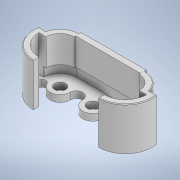
# Autodesk Inventor part: Real bottom
Saved by Autodesk Inventor 2020 (Build 240168000, 168)
## iProperties
Created: 2020-02-07
Part Number: Real bottom
Material: Generic
Document SubType Name: Modeling
Designer: Ball
Density: 1 g/cm^3
Appearance: Default
Author: Ball
Autodesk Inventor part; units mm, degrees
ref_plane "YZ Plane" through (0, 0, 0) normal (1, 0, 0) x (0, 1, 0)
ref_plane "XZ Plane" through (0, 0, 0) normal (0, 1, 0) x (-1, 0, 0)
ref_plane "XY Plane" through (0, 0, 0) normal (0, 0, 1) x (1, 0, 0)
sketch "Sketch1" plane through (0, 0, 0) normal (0, 1, 0) x (-1, 0, 0)
  line L0 (-25.6286, 14.9729) -> (-25.6286, 19.0115)
  line L1 (22.987, 19.0115) -> (22.987, 14.9729)
  arc A0 (-36.0426, -0.7751) -> (-25.6286, -11.1891) centre (-25.6286, -0.7751) ccw
  arc A1 (-39.8599, -4.3819) -> (-25.6286, -15.4563) centre (-25.6286, -0.7751) ccw
  line L2 (-25.6286, 14.9729) -> (-25.6286, 16.7446)
  arc A2 (22.987, -11.1891) -> (33.401, -0.7751) centre (22.987, -0.7751) ccw
  arc A3 (22.987, -15.4563) -> (37.2183, -4.3819) centre (22.987, -0.7751) ccw
  line L3 (22.987, 14.9729) -> (22.987, 16.7446)
  line L4 (-36.0426, -0.7751) -> (-41.3766, -0.7751)
  line L5 (-45.1939, -4.3446) -> (-45.1939, -4.3819)
  line L6 (-45.1939, -4.3819) -> (-39.8599, -4.3819)
  line L7 (33.401, -0.7751) -> (38.735, -0.7751)
  line L8 (42.5523, -4.3819) -> (37.2183, -4.3819)
  arc A4 (-25.6286, 14.9729) -> (-41.3766, -0.7751) centre (-25.6286, -0.7751) ccw
  line L9 (37.2183, -4.3819) -> (42.5523, -4.3819)
  line L10 (42.5523, -4.3819) -> (42.5523, -4.3446)
  line L11 (42.5523, -4.3819) -> (42.5523, -4.3446)
  arc A5 (-25.6286, 19.1131) -> (-45.187, -4.3819) centre (-25.6286, -0.7751) ccw
  line L12 (-25.6286, 14.9729) -> (-25.6286, 19.1131)
  arc A6 (38.735, -0.7751) -> (22.987, 14.9729) centre (22.987, -0.7751) ccw
  line L13 (22.987, 14.9729) -> (22.987, 19.1131)
  arc A7 (42.5454, -4.3819) -> (22.987, 19.1131) centre (22.987, -0.7751) ccw
  line L14 (22.987, -12.3321) -> (-25.6286, -12.3321)
  line L15 (-25.6286, -11.1891) -> (-25.6286, -12.3321)
  line L16 (-25.6286, -15.4563) -> (-25.6286, -16.5993)
  line L17 (22.987, -15.4563) -> (22.987, -16.5993)
  line L18 (22.987, -11.1891) -> (22.987, -12.3321)
  line L19 (22.987, -16.5993) -> (-25.6286, -16.5993)
  point P0 (0, 0)
  dimension "d19" = 15.748
  dimension "d20" = 31.496
  dimension "d21" = 19.8882
  dimension "d38" = 5.334
  dimension "d39" = 5.334
  dimension "d40" = 14.6812
  dimension "d41" = 10.414
  dimension "d45" = 10.414
  dimension "d46" = 14.6812
  dimension "d47" = 19.8882
  dimension "d48" = 5.334
  dimension "d49" = 5.334
  dimension "d50" = 4.0386
  dimension "d51" = 4.0386
  dimension "d55" = 1.143
  dimension "d56" = 1.143
  dimension "d57" = 4.2672
  dimension "d58" = 1.143
  dimension "d59" = 1.143
  dimension "d61" = 48.6156
  constraints: 40 end point, 18 point on circle, 8 centre point, 6 coincident, 5 horizontal, 5 point on line, 5 vertical, 3 parallel, 2 perpendicular
  measures "d19" radius of A4
  measures "d20" diameter of A6
  measures "d21" radius of A5
  measures "d38" distance of L5.end L6.end
  measures "d39" distance of L4.start L4.end
  measures "d40" radius of A1
  measures "d41" radius of A0
  measures "d45" radius of A2
  measures "d46" radius of A3
  measures "d47" radius of A7
  measures "d48" distance of L8.start L8.end
  measures "d49" distance of L7.start L7.end
  measures "d50" distance of L1.start L1.end
  measures "d51" distance of L0.start L0.end
  measures "d55" distance of L16.start L16.end
  measures "d56" distance of L17.start L17.end
  measures "d57" distance between parallel lines of L14 L19
  measures "d58" distance of L15.start L14.end
  measures "d59" distance of L18.start L14.start
  measures "d61" distance of A0.centre A2.centre
extrude "Extrusion1" add sketch "Sketch1" along normal blind 31.9278 contours A4 L4 A0 L15 L14 L18 A2 L7 A6 L1 L13 A7 L8 A3 L17 L19 L16 A1 L6 A5 L12 L0
fillet "Fillet1" radius 0.508 6 edges at (34.6448, 31.9278, -12.3615) (42.5234, 31.9278, -4.3819) (40.9138, 31.9278, 11.9491) (-32.0032, 31.9278, -12.3615) (-39.8818, 31.9278, -4.3819) (-38.2722, 31.9278, 11.9491)
sketch "Sketch3" plane through (0, 0, 0) normal (0, 1, 0) x (-1, 0, 0)
  arc A0 (38.735, -0.7751) -> (22.987, 14.9729) centre (22.987, -0.7751) ccw projected
  arc A1 (29.7688, 2.1644) -> (15.5956, -0.7751) centre (22.987, -0.7751) ccw
  arc A2 (6.0706, -0.7751) -> (-8.7122, -0.7751) centre (-1.3208, -0.7751) ccw
  arc A3 (-25.6286, 14.9729) -> (-41.3766, -0.7751) centre (-25.6286, -0.7751) ccw projected
  arc A4 (-18.2372, -0.7751) -> (-32.3901, 2.2108) centre (-25.6286, -0.7751) ccw
  arc A5 (6.0706, -0.7751) -> (15.5956, -0.7751) centre (10.8331, -0.7751) ccw
  arc A6 (-18.2372, -0.7751) -> (-8.7122, -0.7751) centre (-13.4747, -0.7751) ccw
  circle A7 centre (22.987, -0.7751) radius 4.064
  circle A8 centre (-1.3208, -0.7751) radius 4.064
  circle A9 centre (-25.6286, -0.7751) radius 4.064
  line L0 (22.987, 3.2889) -> (22.987, -0.0385)
  arc A10 (29.7688, 2.1644) -> (34.5869, 1.6252) centre (32.3323, 3.2755) ccw
  arc A11 (-37.2512, 1.7608) -> (-32.3901, 2.2108) centre (-34.9459, 3.3395) ccw
  arc A12 (-25.6286, 14.9729) -> (-41.3766, -0.7751) centre (-25.6286, -0.7751) ccw projected
  arc A13 (-37.2829, 9.8163) -> (-37.1522, 1.6252) centre (-31.5598, 5.811) ccw
  arc A14 (34.5869, 1.6252) -> (34.7846, 9.6565) centre (28.973, 5.7815) ccw
  arc A15 (22.987, -15.4563) -> (37.2183, -4.3819) centre (22.987, -0.7751) ccw projected
  arc A16 (22.987, -15.4563) -> (37.2183, -4.3819) centre (22.987, -0.7751) ccw
  line L1 (37.2183, -4.3819) -> (42.5454, -4.3819)
  line L2 (22.987, -15.4563) -> (22.987, -14.9483) projected
  line L3 (22.987, -15.4563) -> (22.987, -16.5993)
  line L4 (22.987, -16.5993) -> (-25.6286, -16.5993)
  arc A17 (-39.8599, -4.3819) -> (-25.6286, -15.4563) centre (-25.6286, -0.7751) ccw projected
  line L5 (-25.6286, -16.5993) -> (-25.6286, -15.4563)
  line L6 (34.7846, 9.6565) -> (39.9199, 9.6565)
  arc A18 (42.5454, -4.3819) -> (22.987, 19.1131) centre (22.987, -0.7751) ccw projected
  arc A19 (42.4387, -4.3819) -> (39.7965, 9.6565) centre (22.987, -0.7751) ccw
  arc A20 (-39.8599, -4.3819) -> (-25.6286, -15.4563) centre (-25.6286, -0.7751) ccw
  line L7 (-45.187, -4.3819) -> (-39.8599, -4.3819) projected
  line L8 (-39.8599, -4.3819) -> (-45.187, -4.3819)
  arc A21 (-42.3882, 9.8163) -> (-45.1235, -4.3819) centre (-25.6286, -0.7751) ccw
  line L9 (-37.2829, 9.8163) -> (-42.3882, 9.8163)
  point P0 (0, 0)
  point P1 (-45.1235, -4.3819)
  dimension "d69" = 8.128
  dimension "d62" = 14.7828
  dimension "d67" = 14.7828
  dimension "d68" = 14.7828
  dimension "d70" = 8.128
  dimension "d71" = 8.128
  dimension "d72" = 3.3274
  dimension "d73" = 5.588
  dimension "d74" = 0
  dimension "d75" = 5.588
  dimension "d76" = 0
  dimension "d77" = 6.985
  constraints: 33 point on circle, 16 end point, 15 centre point, 9 coincident, 7 point on line, 3 horizontal, 2 perpendicular, 2 vertical, 1 collinear, 1 concentric, 1 vertical alignment, 2 other
  measures "d62" diameter of A1
  measures "d67" diameter of A2
  measures "d68" diameter of A4
  measures "d70" diameter of A8
  measures "d71" diameter of A9
  measures "d72" distance of L0.start L0.end
  measures "d73" diameter of A10
  measures "d75" diameter of A11
  measures "d77" radius of A14
extrude "Extrusion2" add sketch "Sketch3" along normal blind 5.0038
sketch "Sketch5" plane through (0, 5.0038, 0) normal (0, 1, 0) x (1, 0, 0)
  circle A0 centre (-22.987, 0.7751) radius 4.064 projected
  arc A1 (-22.987, 12.9671) -> (-10.795, 0.7751) centre (-22.987, 0.7751) ccw
  arc A2 (13.4366, 0.7751) -> (25.6286, 12.9671) centre (25.6286, 0.7751) ccw
  line L0 (-22.987, 11.1891) -> (-22.987, 12.3321) projected
  line L1 (-10.795, 0.7751) -> (13.4366, 0.7751)
  line L2 (25.6286, 12.3321) -> (25.6286, 11.1891) projected
  line L3 (-22.987, 12.9671) -> (25.6286, 12.9671)
  point P0 (0, 0)
  dimension "d80" = 24.384
  dimension "d81" = 24.384
  constraints: 4 end point, 4 point on circle, 2 centre point, 2 horizontal, 1 coincident
  measures "d80" diameter of A1
  measures "d81" diameter of A2
extrude "Extrusion3" cut sketch "Sketch5" along normal blind 6.35
fillet "Fillet2" radius 0.508 9 edges at (1.3208, 11.3538, -12.3321) (-30.3508, 11.3538, -8.1389) (-34.29, 11.3538, -0.7751) (-22.987, 11.3538, -11.7606) (25.6286, 11.3538, -11.7606) (32.9924, 11.3538, -8.1389) (36.9316, 11.3538, -0.7751) (37.8206, 8.1788, -0.7751) (-35.179, 8.1788, -0.7751)
body "Solid1"
